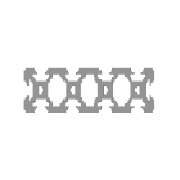
# Autodesk Inventor part: vslot 20 x 80
Saved by Autodesk Inventor 2013 (Build 170138000, 138)
## iProperties
Created: 2013-12-08
Part Number: vslot 20 x 80
Material: Aluminum 6061
Document SubType Name: Modeling
Standard: Unnamed
Designer: Work
Language: en-US
Size Designation: vslot 20 x 80
Categories: <MemberInstance><Categories><Category DisplayName="Structural Shapes" InternalName="089c4875-fa83-4c05-b084-43b9cc11f5ed" Mnemonic="GRDR"><CategoryParameter DisplayName="Custom Base Point" InternalName="4f1d1b73-316d-484b-a3df-9cbabb16eb77" Mnemonic="shpBasePoint"/><CategoryParameter DisplayName="FG Authored" InternalName="9c666724-f362-4ea7-ac62-f6a007de5c69" Mnemonic="shpFGAuto"/><CategoryParameter DisplayName="Legacy Member ID" InternalName="340afe4f-75d7-48d3-ab7d-943f3c3da468" Mnemonic="LegacyMemberID"/><CategoryParameter DisplayName="Base Length" InternalName="42e34263-8f20-4d0e-ad48-bf1385b87c24" Mnemonic="shplen"/><CategoryParameter DisplayName="Distance of the Center of Gravity X-X" InternalName="26c9bdb8-9c79-4b4f-a92e-8e197583c9c4" Mnemonic="grcendistX"/><CategoryParameter DisplayName="Distance of the Center of Gravity Y-Y" InternalName="bcc4fb17-7af4-436a-8f8c-d0aa3b0248c5" Mnemonic="grcendistY"/><CategoryParameter DisplayName="Torsional Rigidity Modulus" InternalName="26c1ec35-5026-4c63-ad0a-751cf684a536" Mnemonic="torrigmod"/><CategoryParameter DisplayName="Torsional Section Modulus" InternalName="7c55a8dc-8844-49f9-a867-cc677b30ec9a" Mnemonic="torsecmod"/><CategoryParameter DisplayName="Coefficient of Shear Displacement" InternalName="de4c90c6-aaa8-468f-a335-6737b311b5d3" Mnemonic="shdispc"/><CategoryParameter DisplayName="Section Area" InternalName="1ff91680-64b0-4202-b9a3-7fd3f94bba3b" Mnemonic="secarea"/><CategoryParameter DisplayName="Moment of Inertia (x)" InternalName="4cd780bc-73d7-43ac-917a-579e5cbd684d" Mnemonic="inermomx"/><CategoryParameter DisplayName="Moment of Inertia (y)" InternalName="4b9f58ea-bced-460e-81ea-3d29ca5a49e3" Mnemonic="inermomy"/><CategoryParameter DisplayName="Section Module (x)" InternalName="72cfad18-cf51-4ed4-aaa7-c6b224f8419f" Mnemonic="secmodx"/><CategoryParameter DisplayName="Section Module (y)" InternalName="59eaa5e9-d227-48dc-b6c1-6920f96e0f95" Mnemonic="secmody"/><CategoryParameter DisplayName="Radius of Gyration (x)" InternalName="25778675-03e9-40c1-b6a8-4a9ed693320d" Mnemonic="gyrradx"/><CategoryParameter DisplayName="Radius of Gyration (y)" InternalName="bfa18ebe-1636-4dbe-8d42-b263e0b73184" Mnemonic="gyrrady"/><CategoryParameter DisplayName="Shape Thickness" InternalName="d109cf76-8eb4-42fc-9800-4409734adc67" Mnemonic="shpthick"/><CategoryParameter DisplayName="Second Shape Thickness" InternalName="9251a8e1-85fd-4e47-af99-afdb762317d9" Mnemonic="shpthick2"/><CategoryParameter DisplayName="Shape Width" InternalName="7c717d54-a18f-4666-b4d4-573cce22c62c" Mnemonic="shpwdth"/><CategoryParameter DisplayName="Shape Height" InternalName="50274e7d-5ac0-4796-92cb-c59e54983c67" Mnemonic="shpheig"/><CategoryParameter DisplayName="Mass per Length Unit" InternalName="0bb95a10-148f-4027-a459-38d7b056702a" Mnemonic="shpmass"/><CategoryParameter DisplayName="Section Designation" InternalName="5a64d034-428d-49c8-ba32-7619764de20f" Mnemonic="shpdes"/><Category DisplayName="Square/Rectangular Tubes" InternalName="afc8e2d8-05d6-4609-8807-f98a9b7d2ed0" Mnemonic="SQRSHP"><CategoryParameter DisplayName="Moment of Inertia (x)" InternalName="8c4637b6-6b69-4878-9d5d-26a32185d655" Mnemonic="inermomx"/><CategoryParameter DisplayName="Moment of Inertia (y)" InternalName="55ec8510-8276-4c45-8f10-594e0fee7eb3" Mnemonic="inermomy"/><CategoryParameter DisplayName="Section Module (x)" InternalName="50d965a6-04bf-46b9-8ace-861858d348e6" Mnemonic="secmodx"/><CategoryParameter DisplayName="Section Module (y)" InternalName="5106aeac-54a2-4159-a9af-8933dd39dba2" Mnemonic="secmody"/><CategoryParameter DisplayName="Section Area" InternalName="2f7f79dd-983c-4263-802a-5b6a1495fdc5" Mnemonic="secarea"/><CategoryParameter DisplayName="Radius of Gyration (x)" InternalName="56c89926-a299-4389-a862-ac94c9691272" Mnemonic="gyrradx"/><CategoryParameter DisplayName="Radius of Gyration (y)" InternalName="fa48a7f5-f030-40f9-a60b-de8a845b7104" Mnemonic="gyrrady"/><CategoryParameter DisplayName="Shape Width" InternalName="8c8a1782-5e80-4d77-858b-304b1c0ad1fd" Mnemonic="shpwdth"/><CategoryParameter DisplayName="Shape Thickness" InternalName="52712fc5-f4ee-4eda-b3f2-6fce82c26419" Mnemonic="shpthick"/><CategoryParameter DisplayName="Radius" InternalName="5d8d062c-e28e-41c1-98da-8e5fee36da1a" Mnemonic="shprad"/></Category></Category><Category DisplayName="DataType" InternalName="23b78d0f-2648-40c6-8793-ca6db495c9e8" Mnemonic="DATATYPE"><CategoryParameter DisplayName="DisplayName" InternalName="05415f3d-3907-474b-a020-eb9d644f4cf3" Mnemonic="DISPLAYNAME"/><CategoryParameter DisplayName="InternalName" InternalName="cf1d0246-76d9-4b4a-8305-fa0409afb5c1" Mnemonic="INTERNALNAME"/><CategoryParameter DisplayName="Folder Name" InternalName="3f06958e-8713-4116-9be7-ed6184ecc97b" Mnemonic="FOLDERNAME"/><CategoryParameter DisplayName="Family Version" InternalName="914462f6-6e19-4b14-ba84-155b9680b1d0" Mnemonic="FAMILYREVISION"/><CategoryParameter DisplayName="ClipFormat" InternalName="bc51e27b-3422-4e78-93ef-cec197ddf230" Mnemonic="CLIPFORMAT"/><CategoryParameter DisplayName="IsMetric" InternalName="e2385c5b-1ea4-4823-96a8-8de651266ec3" Mnemonic="ISMETRIC"/><CategoryParameter DisplayName="Description" InternalName="13903e3d-64b1-4950-80da-f627842ea37f" Mnemonic="DESCRIPTION"/><CategoryParameter DisplayName="StdsOrg" InternalName="8f5914e1-4693-403f-8ab5-d37768198c9d" Mnemonic="STDSORG"/><CategoryParameter DisplayName="Standard" InternalName="0c0a119c-1e12-4c84-803f-101930972f5e" Mnemonic="STANDARD"/><CategoryParameter DisplayName="Manufacturer" InternalName="cd6c7a72-a28a-4e50-99a9-2c7f4e13e5ad" Mnemonic="MANUFACTURER"/><CategoryParameter DisplayName="Member Revision" InternalName="a65d44b9-392f-4f4f-857b-e4b3d54996fe" Mnemonic="MEMBERREVISION"/><CategoryParameter DisplayName="Standard Revision" InternalName="91d5a463-65c2-4fde-b823-3b7fea5e8e17" Mnemonic="STANDARDREVISION"/><CategoryParameter DisplayName="Revision Guid" InternalName="45a75005-10b1-4dfc-8d6d-dfe629f0b93c" Mnemonic="REVISIONGUID"/><CategoryParameter DisplayName="Designation" InternalName="2675968c-4ce5-49e0-a4f5-552d29089031" Mnemonic="DESIGNATION"/><CategoryParameter DisplayName="FileName" InternalName="8b46a4cc-9585-4fed-90c3-899f57e09a73" Mnemonic="FILENAME"/><CategoryParameter DisplayName="Default Row" InternalName="2af9ec52-faaa-4026-b378-f9fa4afca842" Mnemonic="DEFAULTROW"/><Category DisplayName="Part" InternalName="c0e0b642-3bcb-4cc8-9e80-f96d35c4afa4" Mnemonic="PART"><CategoryParameter DisplayName="Material" InternalName="818a152a-d3c3-49ca-80ee-df7d91421b8e" Mnemonic="MATERIAL"/><CategoryParameter DisplayName="Material Key" InternalName="5c9a8adb-dd2b-4535-b97f-0a94a95fe41f" Mnemonic="MATERIALKEY"/><CategoryParameter DisplayName="Part Number" InternalName="016b6077-bfbe-49bd-92c9-d8d59c39c941" Mnemonic="PARTNUMBER"/><CategoryParameter DisplayName="Stock Number" InternalName="4dba7c1c-e26c-444e-836c-b08b433409a8" Mnemonic="STOCKNUMBER"/></Category></Category></Categories><FamilyTemplate Id="vslot 20 x 80"><FamilyTemplateParameters><FamilyTemplateParameter ObjectType="kModelParameterObject" ValueType="xs:double" Id="12" ObjectReferenceKey="Length"/><FamilyTemplateParameter ObjectType="kPartComponentDefinitionObject" ValueType="xs:string" Id="23" SubObjectId="Material"/><FamilyTemplateParameter ObjectType="kPropertyObject" ValueType="xs:string" Id="26" ObjectReferenceKey="{32853F0F-3444-11d1-9E93-0060B03C1CA6}" SubObjectId="5"/><FamilyTemplateParameter ObjectType="kPropertyObject" ValueType="xs:string" Id="27" ObjectReferenceKey="{32853F0F-3444-11d1-9E93-0060B03C1CA6}" SubObjectId="52"/></FamilyTemplateParameters></FamilyTemplate><CategoryParameterMap><ParamToTemplateMap><ParamToTemplate CategoryParameter="//CategoryParameter[@InternalName='cf1d0246-76d9-4b4a-8305-fa0409afb5c1']" ConstantValue="ebf7ea96-eb67-4ca1-8d63-a2adbf63b69a"/><ParamToTemplate CategoryParameter="//CategoryParameter[@InternalName='45a75005-10b1-4dfc-8d6d-dfe629f0b93c']" ConstantValue="0c2f275d-c3f9-4ede-bd8e-dbafe7b05320"/><ParamToTemplate CategoryParameter="//CategoryParameter[@InternalName='3f06958e-8713-4116-9be7-ed6184ecc97b']" ConstantValue="vslot 20 x 80"/><ParamToTemplate CategoryParameter="//CategoryParameter[@InternalName='8f5914e1-4693-403f-8ab5-d37768198c9d']" TemplateParameter="17"/><ParamToTemplate CategoryParameter="//CategoryParameter[@InternalName='0c0a119c-1e12-4c84-803f-101930972f5e']" TemplateParameter="18"/><ParamToTemplate CategoryParameter="//CategoryParameter[@InternalName='91d5a463-65c2-4fde-b823-3b7fea5e8e17']" TemplateParameter="19"/><ParamToTemplate CategoryParameter="//CategoryParameter[@InternalName='cd6c7a72-a28a-4e50-99a9-2c7f4e13e5ad']" TemplateParameter="20"/><ParamToTemplate CategoryParameter="//CategoryParameter[@InternalName='13903e3d-64b1-4950-80da-f627842ea37f']" TemplateParameter="22"/><ParamToTemplate CategoryParameter="//CategoryParameter[@InternalName='05415f3d-3907-474b-a020-eb9d644f4cf3']" ConstantValue="vslot 20 x 80"/><ParamToTemplate CategoryParameter="//CategoryParameter[@InternalName='914462f6-6e19-4b14-ba84-155b9680b1d0']" ConstantValue="11"/><ParamToTemplate CategoryParameter="//CategoryParameter[@InternalName='bc51e27b-3422-4e78-93ef-cec197ddf230']" ConstantValue="CF_INVENTOR.STDPARTS"/><ParamToTemplate CategoryParameter="//CategoryParameter[@InternalName='e2385c5b-1ea4-4823-96a8-8de651266ec3']" ConstantValue="true"/><ParamToTemplate CategoryParameter="//CategoryParameter[@InternalName='2af9ec52-faaa-4026-b378-f9fa4afca842']" ConstantValue="1"/><ParamToTemplate CategoryParameter="//CategoryParameter[@InternalName='9c666724-f362-4ea7-ac62-f6a007de5c69']" ConstantValue="1"/><ParamToTemplate CategoryParameter="//CategoryParameter[@InternalName='8b46a4cc-9585-4fed-90c3-899f57e09a73']" ConstantValue="vslot 20 x 80-10"/><ParamToTemplate CategoryParameter="//CategoryParameter[@InternalName='a65d44b9-392f-4f4f-857b-e4b3d54996fe']" ConstantValue="1856a6cc-7cb3-40a6-bba1-c2a638bcb572"/><ParamToTemplate CategoryParameter="//CategoryParameter[@InternalName='a65d44b9-392f-4f4f-857b-e4b3d54996fe']" ConstantValue="1856a6cc-7cb3-40a6-bba1-c2a638bcb572"/><ParamToTemplate CategoryParameter="//CategoryParameter[@InternalName='2675968c-4ce5-49e0-a4f5-552d29089031']" TemplateParameter="27"/><ParamToTemplate CategoryParameter="//CategoryParameter[@InternalName='42e34263-8f20-4d0e-ad48-bf1385b87c24']" TemplateParameter="12"/><ParamToTemplate CategoryParameter="//CategoryParameter[@InternalName='818a152a-d3c3-49ca-80ee-df7d91421b8e']" TemplateParameter="23"/><ParamToTemplate CategoryParameter="//CategoryParameter[@InternalName='016b6077-bfbe-49bd-92c9-d8d59c39c941']" TemplateParameter="26"/></ParamToTemplateMap></CategoryParameterMap></MemberInstance>
Mass: 15.0002 g
Surface Area: 68.3855 cm^2
Volume: 5.53512 cm^3
Density: 2.71 g/cm^3
_CCFamilyDisplayName: vslot 20 x 80
_FrameMemberDoc: Frame Member File
_Version: 15.0.0
_GetPNFromCC: 1
G_L: 475.000 mm
G_W: 80.000 mm
G_H: 20.000 mm
IsCustomPart: 1
Author: Work
Autodesk Inventor part; units mm, degrees
ref_plane "YZ Plane" through (0, 0, 0) normal (1, 0, 0) x (0, 1, 0)
ref_plane "XZ Plane" through (0, 0, 0) normal (0, 1, 0) x (-1, 0, 0)
ref_plane "Start Plane" through (0, 0, 0) normal (0, 0, 1) x (1, 0, 0)
ref_plane "End Plane" through (0, 0, 475) normal (0, 0, 1) x (1, 0, 0)
sketch "Sketch" plane through (0, 0, 0) normal (0, 0, 1) x (1, 0, 0)
  line L0 (0, 0) -> (0, 10) construction
  line L1 (0, 10) -> (-10, 10) construction
  line L2 (-10, 10) -> (-10, 0) construction
  line L3 (-10, 10) -> (-20, 10) construction
  line L4 (-20, 10) -> (-20, 0) construction
  circle A0 centre (-10, 0) radius 2.1
  line L5 (-13.9007, -3.9007) -> (-6.0993, -3.9007) construction
  line L6 (-6.0993, -3.9007) -> (-6.0993, 3.9007) construction
  line L7 (-6.0993, 3.9007) -> (-13.9007, 3.9007) construction
  line L8 (-13.9007, 3.9007) -> (-13.9007, -3.9007) construction
  line L9 (-13.9007, -3.9007) -> (-6.0993, 3.9007) construction
  line L10 (-6.0993, -3.9007) -> (-13.9007, 3.9007) construction
  line L11 (-13.9007, -2.84) -> (-12.84, -3.9007) construction
  line L12 (-13.9007, -2.84) -> (-12.4007, -2.84) construction
  line L13 (0, 0) -> (-10, 0) construction
  line L14 (-12.84, -3.9007) -> (-15.4993, -6.56)
  line L15 (-15.4993, -6.56) -> (-15.4993, -8.2)
  line L16 (-15.4993, -8.2) -> (-12.84, -8.2)
  line L17 (-12.84, -8.2) -> (-14.64, -10)
  line L18 (-7.16, -3.9007) -> (-4.5007, -6.56)
  line L19 (-4.5007, -6.56) -> (-4.5007, -8.2)
  line L20 (-4.5007, -8.2) -> (-7.16, -8.2)
  line L21 (-7.16, -8.2) -> (-5.36, -10)
  line L22 (-12.84, 3.9007) -> (-15.4993, 6.56)
  line L23 (-15.4993, 6.56) -> (-15.4993, 8.2)
  line L24 (-15.4993, 8.2) -> (-12.84, 8.2)
  line L25 (-12.84, 8.2) -> (-14.64, 10)
  line L26 (-7.16, 3.9007) -> (-4.5007, 6.56)
  line L27 (-4.5007, 6.56) -> (-4.5007, 8.2)
  line L28 (-4.5007, 8.2) -> (-7.16, 8.2)
  line L29 (-7.16, 8.2) -> (-5.36, 10)
  line L30 (-20, -8.2) -> (-15.4993, -8.2) construction
  line L31 (-13.9007, -2.84) -> (-17.3007, -6.24)
  line L32 (-17.3007, -6.24) -> (-17.3007, -8.2)
  line L33 (-13.9007, 2.84) -> (-17.3007, 6.24)
  line L34 (-17.3007, 6.24) -> (-17.3007, 8.2)
  line L35 (-6.0993, -2.84) -> (-2.6993, -6.24)
  line L36 (-2.6993, -6.24) -> (-2.6993, -8.2)
  line L37 (-2.6993, 6.24) -> (-2.6993, 8.2)
  line L38 (-6.0993, 2.84) -> (-2.6993, 6.24)
  line L39 (-12.84, -3.9007) -> (-7.16, -3.9007)
  line L40 (-6.0993, -2.84) -> (-6.0993, 2.84)
  line L41 (-7.16, 3.9007) -> (-12.84, 3.9007)
  line L42 (-13.9007, 2.84) -> (-13.9007, -2.84)
  line L43 (-30, 10) -> (-30, 0) construction
  circle A1 centre (-30, 0) radius 2.1
  line L44 (-26.0993, -3.9007) -> (-33.9007, -3.9007) construction
  line L45 (-33.9007, -3.9007) -> (-33.9007, 3.9007) construction
  line L46 (-33.9007, 3.9007) -> (-26.0993, 3.9007) construction
  line L47 (-26.0993, 3.9007) -> (-26.0993, -3.9007) construction
  line L48 (-26.0993, -3.9007) -> (-33.9007, 3.9007) construction
  line L49 (-33.9007, -3.9007) -> (-26.0993, 3.9007) construction
  line L50 (-26.0993, -2.84) -> (-27.16, -3.9007) construction
  line L51 (-26.0993, -2.84) -> (-27.5993, -2.84) construction
  line L52 (-27.16, -3.9007) -> (-24.5007, -6.56)
  line L53 (-24.5007, -6.56) -> (-24.5007, -8.2)
  line L54 (-24.5007, -8.2) -> (-27.16, -8.2)
  line L55 (-27.16, -8.2) -> (-25.36, -10)
  line L56 (-32.84, -3.9007) -> (-35.4993, -6.56)
  line L57 (-35.4993, -6.56) -> (-35.4993, -8.2)
  line L58 (-35.4993, -8.2) -> (-32.84, -8.2)
  line L59 (-32.84, -8.2) -> (-34.64, -10)
  line L60 (-27.16, 3.9007) -> (-24.5007, 6.56)
  line L61 (-24.5007, 6.56) -> (-24.5007, 8.2)
  line L62 (-24.5007, 8.2) -> (-27.16, 8.2)
  line L63 (-27.16, 8.2) -> (-25.36, 10)
  line L64 (-32.84, 8.2) -> (-34.64, 10)
  line L65 (-35.4993, 8.2) -> (-32.84, 8.2)
  line L66 (-35.4993, 6.56) -> (-35.4993, 8.2)
  line L67 (-32.84, 3.9007) -> (-35.4993, 6.56)
  line L68 (-26.0993, -2.84) -> (-22.6993, -6.24)
  line L69 (-22.6993, -6.24) -> (-22.6993, -8.2)
  line L70 (-22.6993, 6.24) -> (-22.6993, 8.2)
  line L71 (-26.0993, 2.84) -> (-22.6993, 6.24)
  line L72 (-27.16, -3.9007) -> (-32.84, -3.9007)
  line L73 (-33.9007, -2.84) -> (-33.9007, 2.84)
  line L74 (-32.84, 3.9007) -> (-27.16, 3.9007)
  line L75 (-26.0993, 2.84) -> (-26.0993, -2.84)
  line L76 (-38.2, -2.84) -> (-40, -4.64)
  line L77 (-36.56, -5.4993) -> (-38.2, -5.4993)
  line L78 (-38.2, -5.4993) -> (-38.2, -2.84)
  line L79 (-33.9007, -2.84) -> (-36.56, -5.4993)
  line L80 (-33.9007, 2.84) -> (-36.56, 5.4993)
  line L81 (-36.56, 5.4993) -> (-38.2, 5.4993)
  line L82 (-38.2, 2.84) -> (-40, 4.64)
  line L83 (-38.2, 5.4993) -> (-38.2, 2.84)
  line L84 (10, 10) -> (10, 0) construction
  line L85 (10, 10) -> (20, 10) construction
  line L86 (20, 10) -> (20, 0) construction
  circle A2 centre (10, 0) radius 2.1
  line L87 (13.9007, -3.9007) -> (6.0993, -3.9007) construction
  line L88 (6.0993, -3.9007) -> (6.0993, 3.9007) construction
  line L89 (6.0993, 3.9007) -> (13.9007, 3.9007) construction
  line L90 (13.9007, 3.9007) -> (13.9007, -3.9007) construction
  line L91 (13.9007, -3.9007) -> (6.0993, 3.9007) construction
  line L92 (6.0993, -3.9007) -> (13.9007, 3.9007) construction
  line L93 (13.9007, -2.84) -> (12.84, -3.9007) construction
  line L94 (13.9007, -2.84) -> (12.4007, -2.84) construction
  line L95 (12.84, -3.9007) -> (15.4993, -6.56)
  line L96 (15.4993, -6.56) -> (15.4993, -8.2)
  line L97 (15.4993, -8.2) -> (12.84, -8.2)
  line L98 (12.84, -8.2) -> (14.64, -10)
  line L99 (7.16, -3.9007) -> (4.5007, -6.56)
  line L100 (4.5007, -6.56) -> (4.5007, -8.2)
  line L101 (4.5007, -8.2) -> (7.16, -8.2)
  line L102 (7.16, -8.2) -> (5.36, -10)
  line L103 (12.84, 3.9007) -> (15.4993, 6.56)
  line L104 (15.4993, 6.56) -> (15.4993, 8.2)
  line L105 (15.4993, 8.2) -> (12.84, 8.2)
  line L106 (12.84, 8.2) -> (14.64, 10)
  line L107 (7.16, 8.2) -> (5.36, 10)
  line L108 (4.5007, 8.2) -> (7.16, 8.2)
  line L109 (4.5007, 6.56) -> (4.5007, 8.2)
  line L110 (7.16, 3.9007) -> (4.5007, 6.56)
  line L111 (20, -8.2) -> (15.4993, -8.2) construction
  line L112 (13.9007, -2.84) -> (17.3007, -6.24)
  line L113 (17.3007, -6.24) -> (17.3007, -8.2)
  line L114 (17.3007, 6.24) -> (17.3007, 8.2)
  line L115 (13.9007, 2.84) -> (17.3007, 6.24)
  line L116 (2.6993, 6.24) -> (2.6993, 8.2)
  line L117 (6.0993, 2.84) -> (2.6993, 6.24)
  line L118 (6.0993, -2.84) -> (2.6993, -6.24)
  line L119 (2.6993, -6.24) -> (2.6993, -8.2)
  line L120 (12.84, -3.9007) -> (7.16, -3.9007)
  line L121 (6.0993, -2.84) -> (6.0993, 2.84)
  line L122 (7.16, 3.9007) -> (12.84, 3.9007)
  line L123 (13.9007, 2.84) -> (13.9007, -2.84)
  line L124 (32.84, 3.9007) -> (35.4993, 6.56)
  line L125 (30, 10) -> (30, 0) construction
  line L126 (35.4993, 6.56) -> (35.4993, 8.2)
  line L127 (35.4993, 8.2) -> (32.84, 8.2)
  line L128 (32.84, 8.2) -> (34.64, 10)
  line L129 (32.84, -8.2) -> (34.64, -10)
  line L130 (35.4993, -6.56) -> (35.4993, -8.2)
  line L131 (35.4993, -8.2) -> (32.84, -8.2)
  line L132 (32.84, -3.9007) -> (35.4993, -6.56)
  line L133 (26.0993, 2.84) -> (26.0993, -2.84)
  line L134 (32.84, 3.9007) -> (27.16, 3.9007)
  line L135 (33.9007, -2.84) -> (33.9007, 2.84)
  line L136 (27.16, -3.9007) -> (32.84, -3.9007)
  line L137 (27.16, 3.9007) -> (24.5007, 6.56)
  line L138 (33.9007, 3.9007) -> (26.0993, 3.9007) construction
  circle A3 centre (30, 0) radius 2.1
  line L139 (26.0993, 3.9007) -> (26.0993, -3.9007) construction
  line L140 (26.0993, -3.9007) -> (33.9007, -3.9007) construction
  line L141 (26.0993, -3.9007) -> (33.9007, 3.9007) construction
  line L142 (33.9007, -3.9007) -> (26.0993, 3.9007) construction
  line L143 (33.9007, -3.9007) -> (33.9007, 3.9007) construction
  line L144 (26.0993, -2.84) -> (27.5993, -2.84) construction
  line L145 (27.16, -8.2) -> (25.36, -10)
  line L146 (26.0993, -2.84) -> (27.16, -3.9007) construction
  line L147 (27.16, -3.9007) -> (24.5007, -6.56)
  line L148 (24.5007, -8.2) -> (27.16, -8.2)
  line L149 (24.5007, -6.56) -> (24.5007, -8.2)
  line L150 (26.0993, -2.84) -> (22.6993, -6.24)
  line L151 (22.6993, -6.24) -> (22.6993, -8.2)
  line L152 (26.0993, 2.84) -> (22.6993, 6.24)
  line L153 (24.5007, 8.2) -> (27.16, 8.2)
  line L154 (24.5007, 6.56) -> (24.5007, 8.2)
  line L155 (22.6993, 6.24) -> (22.6993, 8.2)
  line L156 (27.16, 8.2) -> (25.36, 10)
  line L157 (33.9007, -2.84) -> (36.56, -5.4993)
  line L158 (36.56, -5.4993) -> (38.2, -5.4993)
  line L159 (38.2, -2.84) -> (40, -4.64)
  line L160 (38.2, -5.4993) -> (38.2, -2.84)
  line L161 (33.9007, 2.84) -> (36.56, 5.4993)
  line L162 (36.56, 5.4993) -> (38.2, 5.4993)
  line L163 (38.2, 5.4993) -> (38.2, 2.84)
  line L164 (38.2, 2.84) -> (40, 4.64)
  line L165 (-25.36, -10) -> (-14.64, -10)
  line L166 (-5.36, -10) -> (5.36, -10)
  line L167 (14.64, -10) -> (25.36, -10)
  line L168 (34.64, -10) -> (38, -10)
  line L169 (40, -8) -> (40, -4.64)
  line L170 (40, 4.64) -> (40, 8)
  line L171 (38, 10) -> (34.64, 10)
  line L172 (25.36, 10) -> (14.64, 10)
  line L173 (5.36, 10) -> (-5.36, 10)
  line L174 (-14.64, 10) -> (-25.36, 10)
  line L175 (-34.64, 10) -> (-38, 10)
  line L176 (-40, 8) -> (-40, 4.64)
  line L177 (-40, -4.64) -> (-40, -8)
  line L178 (-38, -10) -> (-34.64, -10)
  line L179 (-22.6993, 8.2) -> (-17.3007, 8.2)
  line L180 (-22.6993, -8.2) -> (-17.3007, -8.2)
  line L181 (-2.6993, 8.2) -> (2.6993, 8.2)
  line L182 (-2.6993, -8.2) -> (2.6993, -8.2)
  line L183 (17.3007, 8.2) -> (22.6993, 8.2)
  line L184 (17.3007, -8.2) -> (22.6993, -8.2)
  arc A4 (-40, -8) -> (-38, -10) centre (-38, -8) ccw
  arc A5 (-38, 10) -> (-40, 8) centre (-38, 8) ccw
  arc A6 (38, -10) -> (40, -8) centre (38, -8) ccw
  arc A7 (40, 8) -> (38, 10) centre (38, 8) ccw
  dimension "d0" = 10
  dimension "d1" = 10
  dimension "d2" = 10
  dimension "d3" = 4.2
  dimension "d4" = 1.5
  dimension "d5" = 45
  dimension "d6" = 1.64
  dimension "d7" = 1.8
  dimension "d8" = 10
  dimension "d9" = 2.84
  dimension "d11" = 135
  dimension "d12" = 1.96
  dimension "d13" = 5.68
  dimension "d14" = 2
  constraints: 370 end point, 155 symmetric about line, 16 perpendicular, 13 collinear, 11 point on line, 10 parallel, 8 centre point, 8 midpoint, 8 point on circle, 8 tangent, 4 coincident, 3 equal radius, 2 horizontal, 1 equal length, 1 vertical, 3 other
  measures "d0" distance of L0.start L0.end
  measures "d1" distance of L0.end L1.end
  measures "d2" distance of L1.end L3.end
  measures "d3" diameter of A0
  measures "d4" distance of L11.start L11.end
  measures "d5" angle of L11 L12
  measures "d6" distance of L14.end L15.end
  measures "d7" horizontal distance of L16.end L17.end
  measures "d8" vertical distance of L2.end L17.end
  measures "d9" distance from line of L11.end L2
  measures "d11" angle of L8 L31
  measures "d12" distance of L31.end L32.end
  measures "d13" distance of L20.end L16.end
  measures "d14" radius of A4
extrude "Body" add sketch "Sketch" along normal up to surface (475 mm away) from surface at 0
sketch "Sketch10" plane through (0, 0, 0) normal (0, 0, 1) x (1, 0, 0)
  line L0 (0, 0) -> (10, 0)
ref_plane "Work Plane7" through (0, 0, 0) normal (0, -1, 0) x (1, 0, 0)
sketch "Sketch11" plane through (0, 0, 0) normal (0, -1, 0) x (1, 0, 0)
  line L0 (-2, 0) -> (12, 0)
  line L1 (-2, 475) -> (12, 475)
  dimension "d22" = 475
  measures "d22" distance between parallel lines of L0 L1
equation "\"G_OFFSET_START\" = 0"
equation "\"G_OFFSET_END\" = 0"
equation "\"d18\" = Length + G_OFFSET_END"
equation "\"G_L\" = d22"
equation "\"Length\" = 475"
body "Solid1"
